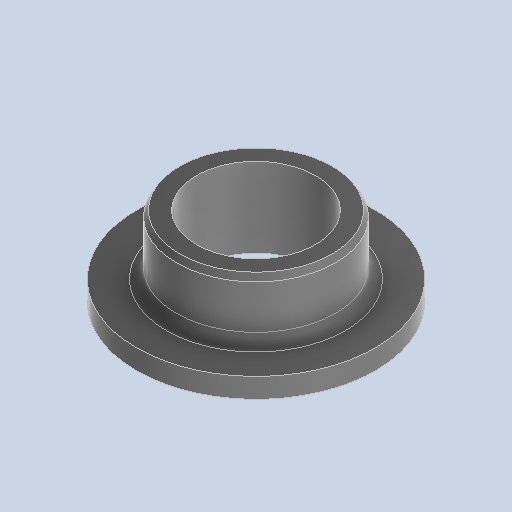
# Autodesk Inventor part: GFM-0608-04
Saved by Autodesk Inventor 2024.2 (Build 282272000, 272)
## iProperties
Part Number: GFM-0608-04
Material: Acetal Resin, Black
Document SubType Name: Modeling
Designer: Masato Kubotera
Density: 1.425 g/cm^3
Appearance: Smooth - Black
Catalog Web Link: https://jp.misumi-ec.com/vona2/detail/221000103492/?ProductCode=GFM-0608-04
Vendor: igus
Mass: 0.207149 g
Surface Area: 3.44616 cm^2
Volume: 0.145368 cm^3
Author: Masato Kubotera
Autodesk Inventor part; units mm, degrees
ref_plane "YZ Plane" through (0, 0, 0) normal (1, 0, 0) x (0, 1, 0)
ref_plane "XZ Plane" through (0, 0, 0) normal (0, 1, 0) x (-1, 0, 0)
ref_plane "XY Plane" through (0, 0, 0) normal (0, 0, 1) x (1, 0, 0)
sketch "Sketch1" plane through (0, 0, 0) normal (0, 1, 0) x (-1, 0, 0)
  line L0 (0, 0) -> (0, 4)
  line L1 (-3, 0) -> (-3, 4)
  line L2 (-3, 4) -> (-4, 4)
  line L3 (-4, 4) -> (-4, 1)
  line L4 (-4, 1) -> (-6, 1)
  line L5 (-6, 1) -> (-6, 0)
  line L6 (-6, 0) -> (-3, 0)
  dimension "InsideDiameter" = 6
  dimension "OuterDiameter" = 8
  dimension "FlangeDiameter" = 12
  dimension "FlangeThickness" = 1
  dimension "Length" = 3
  constraints: 14 end point, 4 vertical, 3 horizontal, 2 point on line
  measures "InsideDiameter" diameter of L1 L0
  measures "OuterDiameter" diameter of L3 L0
  measures "FlangeDiameter" diameter of L5 L0
  measures "FlangeThickness" distance of L4.end L5.end
  measures "Length" distance of L2.end L3.end
revolve "Revolution1" add sketch "Sketch1" angle 360 about axis through (0, 0, 0) along (0, 0, 1)
chamfer "Chamfer1" distance 0.3 angle 30 1 edges at (-4, 0, 4) measured on face at (3.987, -0.3219, 3)
fillet "Fillet1" radius 0.5 1 edges at (-4, 0, 1)
body "Solid1"
